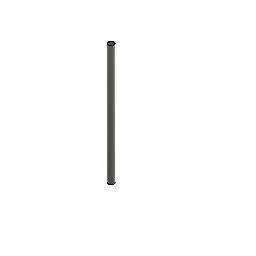
Axis1tube (Autodesk Fusion 360 design; units mm, degrees)
Autodesk Fusion 360 part; units mm, degrees
sketch "Sketch1" plane through (-47, 8, 12) normal (0, 1, 0) x (-1, 0, 0)
  circle A0 centre (-47, -12) radius 6
  circle A1 centre (-47, -12) radius 14
  circle A2 centre (-47, -12) radius 5
  circle A3 centre (-47, -12) radius 6
  dimension "d1039" = 1
  dimension "d1040" = 12
  measures "d1039" distance of A2 A3
  measures "d1040" diameter of A3
extrude "Extrude1" add sketch "Sketch1" along normal blind 3 and the other way up to surface (253 mm away) contours A0 A3
chamfer "Chamfer1" distance 0.5 angle 45 1 edges at (4.6616, 11, 1.8081)
sketch "Sketch2" plane through (69, 0, 0) normal (1, 0, 0) x (0, 0, -1)
  arc A0 (17.1962, -239) -> (6.8038, -239) centre (12, -236) ccw
  line L0 (17.1962, -239) -> (24, -239)
  line L1 (24, -239) -> (24, -219)
  line L2 (24, -219) -> (0, -219)
  line L3 (0, -219) -> (0, -239)
  line L4 (0, -239) -> (6.8038, -239)
  circle A1 centre (12, -236) radius 5
  dimension "d1046" = 10
  measures "d1046" diameter of A1
extrude "Extrude2" cut sketch "Sketch2" along normal up to surface contours A1 end surface at (-4.9938, 9.6667, -0.2492)
sketch "Sketch3" plane through (25, 0, 0) normal (-1, 0, 0) x (0, 0, 1)
  line L0 (-15.5, -239) -> (-15.5, -219)
  line L1 (-15.5, -219) -> (-24, -219)
  line L2 (-24, -219) -> (-24, -239)
  line L3 (-24, -239) -> (-15.5, -239)
  circle A0 centre (-12, -223) radius 1.75
  circle A1 centre (-12, -234) radius 1.75
  line L4 (-60, -219) -> (36, -219)
  arc A2 (-13.75, -224.5) -> (-10.25, -224.5) centre (-12, -224.5) ccw
  dimension "d1049" = 3.5
  dimension "d1050" = 4
  dimension "d1051" = 11
  measures "d1049" diameter of A1
extrude "Extrude3" cut sketch "Sketch3" along normal up to surface contours A0 | A1 end surface at (-4.9938, 9.6667, -0.2492)
